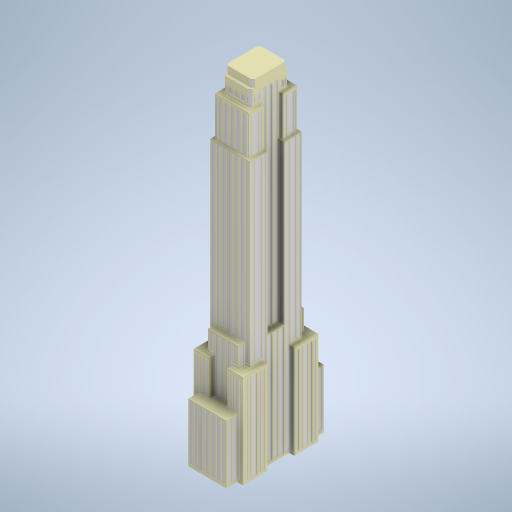
# Autodesk Inventor part: 樓底
Saved by Autodesk Inventor 2024.2 (Build 282272000, 272)
## iProperties
Created: 2024-05-30
Part Number: 樓底
Material: 一般
Document SubType Name: Modeling
Designer: User
Density: 1 g/cm^3
Appearance: 預設
Author: User
Autodesk Inventor part; units mm, degrees
(part 1 of 2)
sketch "草圖2" plane through (0, 0, 0) normal (0, 1, 0) x (-1, 0, 0)
  line L0 (36, 55) -> (36, -55)
  line L1 (36, -55) -> (-36, -55)
  line L2 (-36, -55) -> (-36, 55)
  line L3 (-36, 55) -> (36, 55)
  line L4 (36, 55) -> (-36, -55) construction
  line L5 (36, -55) -> (-36, 55) construction
  line L6 (36, 0) -> (36, -20)
  line L7 (36, 0) -> (36, 20)
  line L8 (36, 20) -> (36, -20)
  line L9 (36, -20) -> (29, -20)
  line L10 (29, -20) -> (29, 20)
  line L11 (29, 20) -> (36, 20)
  line L12 (0, 55) -> (0, -55)
  line L13 (-36, -20) -> (-29, -20)
  line L14 (-29, -20) -> (-29, 20)
  line L15 (-29, 20) -> (-36, 20)
  line L16 (0, 55) -> (13, 55)
  line L17 (0, 55) -> (-13, 55)
  line L18 (13, 55) -> (-13, 55)
  line L19 (-13, 55) -> (-13, 48)
  line L20 (-13, 48) -> (13, 48)
  line L21 (13, 48) -> (13, 55)
  line L22 (13, 0) -> (-13, 0)
  line L23 (-13, -55) -> (-13, -48)
  line L24 (-13, -48) -> (13, -48)
  line L25 (13, -48) -> (13, -55)
  point P0 (0, 0)
  dimension "d0" = 110
  dimension "d1" = 72
  dimension "d2" = 20
  dimension "d3" = 20
  dimension "d4" = 7
  dimension "d7" = 13
  dimension "d8" = 13
  dimension "d9" = 7
  constraints: 52 end point, 8 symmetric about line, 6 parallel, 5 midpoint, 4 point on line, 3 perpendicular, 2 collinear, 1 horizontal, 1 vertical
  measures "d0" distance of L0.start L0.end
  measures "d1" distance of L0.end L1.end
  measures "d2" distance of L6.start L6.end
  measures "d3" distance of L6.start L7.end
  measures "d4" distance of L6.end L9.end
  measures "d7" distance of L12.start L16.end
  measures "d8" distance of L12.start L17.end
  measures "d9" distance of L19.end L17.end
extrude "擠出2" add sketch "草圖2" along normal blind 137 contours L0 L11 L10 L9 L1 L25 L24 L12 L20 L21 L3 | L19 L20 L12 L24 L23 L1 L2 L13 L14 L15 L3
sketch "草圖3" plane through (0, 137, 0) normal (0, 1, 0) x (1, 0, 0)
  point P0 (0, 0)
sketch "草圖4" plane through (0, 137, 0) normal (0, 1, 0) x (1, 0, 0)
  line L0 (-29, -48) -> (29, -48)
  line L1 (29, -48) -> (29, 48)
  line L2 (29, 48) -> (-29, 48)
  line L3 (-29, 48) -> (-29, -48)
  line L4 (-29, -48) -> (29, 48) construction
  line L5 (29, -48) -> (-29, 48) construction
  line L6 (29, 48) -> (22, 48)
  line L7 (22, 48) -> (22, 38)
  line L8 (22, 38) -> (29, 38)
  line L9 (29, 38) -> (29, 48)
  line L10 (-29, 20) -> (-29, -20) projected
  line L11 (-29, 0) -> (29, 0)
  line L12 (0, 48) -> (0, -48)
  line L13 (-22, 48) -> (-22, 38)
  line L14 (-22, 38) -> (-29, 38)
  line L15 (29, 0) -> (-29, 0)
  line L16 (22, -48) -> (22, -38)
  line L17 (22, -38) -> (29, -38)
  line L18 (0, -48) -> (0, 48)
  line L19 (22, -48) -> (22, -38)
  line L20 (22, -38) -> (29, -38)
  line L21 (-22, -48) -> (-22, -38)
  line L22 (-22, -38) -> (-29, -38)
  point P0 (0, 0)
  dimension "d12" = 7
  dimension "d13" = 10
  constraints: 44 end point, 13 symmetric about line, 6 midpoint, 4 parallel, 2 perpendicular, 1 point on line
  measures "d12" distance of L1.end L6.end
  measures "d13" distance of L7.end L6.end
extrude "擠出3" add sketch "草圖4" along normal blind 29 contours L21 L22 L3 L11 L12 L0 | L12 L11 L1 L17 L16 L0 | L12 L2 L7 L8 L1 L11 | L11 L3 L14 L13 L2 L12
sketch "草圖5" plane through (0, 0, 0) normal (0, -1, 0) x (1, 0, 0)
  line L0 (0, -55) -> (28, -55)
  line L1 (36, -55) -> (13, -55) projected
  line L2 (0, -55) -> (-28, -55)
  line L3 (-13, -55) -> (-36, -55) projected
  line L4 (22, -48) -> (-22, -48) projected
  line L5 (13, -48) -> (-13, -48)
  line L6 (-13, -55) -> (-13, -48)
  line L7 (13, -48) -> (13, -55)
  line L8 (28, -55) -> (-28, -55)
  line L9 (-28, -55) -> (-28, -71)
  line L10 (-28, -71) -> (28, -71)
  line L11 (28, -71) -> (28, -55)
  line L12 (29, 38) -> (29, -38) projected
  line L13 (29, 0) -> (-29, 0)
  line L14 (-29, -38) -> (-29, 38) projected
  line L15 (0, 55) -> (-28, 55)
  line L16 (13, 48) -> (-13, 48)
  line L17 (-13, 55) -> (-13, 48)
  line L18 (13, 48) -> (13, 55)
  line L19 (-28, 55) -> (-28, 71)
  line L20 (-28, 71) -> (28, 71)
  line L21 (28, 71) -> (28, 55)
  line L22 (13, 55) -> (0, 55)
  line L23 (28, 55) -> (-28, 55)
  point P0 (0, 0)
  dimension "d16" = 28
  dimension "d17" = 28
  dimension "d18" = 16
  constraints: 38 end point, 9 symmetric about line, 4 point on line, 3 perpendicular, 2 collinear, 2 midpoint, 2 parallel, 1 horizontal
  measures "d16" distance of L0.start L0.end
  measures "d17" distance of L0.start L2.end
  measures "d18" distance of L9.end L2.end
extrude "擠出4" add sketch "草圖5" against normal blind 86
ref_plane "工作平面1" through (-22, 166, 0) normal (0, 0, 1) x (1, 0, 0)
ref_plane "工作平面3" through (0, 0, -55) normal (-1, 0, 0) x (0, 0, 1)
sketch "草圖12" plane through (0, 166, 0) normal (0, 1, 0) x (1, 0, 0)
  line L0 (29, -20) -> (29, 20) projected
  line L1 (29, 0) -> (29, 12)
  line L2 (29, 0) -> (29, -12)
  line L3 (29, -12) -> (29, 12)
  line L4 (29, 12) -> (20, 12)
  line L5 (20, 12) -> (20, -12)
  line L6 (20, -12) -> (29, -12)
  line L7 (0, -6) -> (0, 6)
  line L8 (-29, 0) -> (-29, 12)
  line L9 (-29, 0) -> (-29, -12)
  line L10 (-29, -12) -> (-29, 12)
  line L11 (-29, 12) -> (-20, 12)
  line L12 (-20, 12) -> (-20, -12)
  line L13 (-20, -12) -> (-29, -12)
  line L14 (-29, -38) -> (-29, -12)
  line L15 (-29, -12) -> (29, -12)
  line L16 (29, -12) -> (29, -38)
  line L17 (29, -38) -> (-29, -38)
  line L18 (-29, -20) -> (-36, -20) projected
  line L19 (-22, 38) -> (-29, 38) projected
  line L20 (-29, 12) -> (-29, 38)
  line L21 (-29, 38) -> (29, 38)
  line L22 (29, 38) -> (29, 12)
  line L23 (29, 12) -> (-29, 12)
  line L24 (-20, -12) -> (-20, 12)
  line L25 (-20, 12) -> (20, 12)
  line L26 (20, 12) -> (20, -12)
  line L27 (20, -12) -> (-20, -12)
  point P0 (0, 0)
  dimension "d89" = 12
  dimension "d90" = 12
  dimension "d91" = 9
  constraints: 50 end point, 8 parallel, 7 perpendicular, 6 symmetric about line, 2 point on line, 1 collinear, 1 midpoint, 1 vertical
  measures "d89" distance of L1.start L1.end
  measures "d90" distance of L1.start L2.end
  measures "d91" distance of L4.end L1.end
extrude "擠出9" add sketch "草圖12" along normal blind 232 contours L16 L17 L14 L13 L15 L6 L0 | L15 L12 L23 L5 | L4 L23 L11 L20 L19 L21 L22 L0
sketch "草圖13" plane through (0, 398, 0) normal (0, 1, 0) x (1, 0, 0)
  line L0 (-25, 35) -> (-25, -35)
  line L1 (-25, -35) -> (25, -35)
  line L2 (25, -35) -> (25, 35)
  line L3 (25, 35) -> (-25, 35)
  line L4 (-25, 35) -> (25, -35) construction
  line L5 (-25, -35) -> (25, 35) construction
  line L6 (-25, 0) -> (-20, 0)
  line L7 (-20, 0) -> (-20, -14)
  line L8 (-20, -14) -> (-25, -14)
  line L9 (-25, -14) -> (-25, 0)
  line L10 (-20, 0) -> (-25, 0)
  line L11 (-25, 0) -> (-25, 14)
  line L12 (-25, 14) -> (-20, 14)
  line L13 (-20, 14) -> (-20, 0)
  line L14 (-20, -12) -> (-20, 12) projected
  line L15 (0, 8.1433) -> (0, -10.4531)
  line L16 (-36, 55) -> (-36, 20) projected
  line L17 (25, 0) -> (20, 0)
  line L18 (20, 0) -> (20, -14)
  line L19 (20, -14) -> (25, -14)
  line L20 (25, -14) -> (25, 0)
  line L21 (20, 0) -> (25, 0)
  line L22 (25, 0) -> (25, 14)
  line L23 (25, 14) -> (20, 14)
  line L24 (20, 14) -> (20, 0)
  line L25 (20, -12) -> (20, 12)
  point P0 (0, 0)
  dimension "d94" = 70
  dimension "d95" = 50
  dimension "d96" = 5
  dimension "d97" = 14
  dimension "d98" = 14
  constraints: 48 end point, 8 symmetric about line, 7 parallel, 5 perpendicular, 3 midpoint, 1 vertical
  measures "d94" distance of L0.start L0.end
  measures "d95" distance of L1.end L0.end
  measures "d96" distance of L6.start L6.end
  measures "d97" distance of L6.end L7.end
  measures "d98" distance of L6.start L11.end
extrude "擠出10" add sketch "草圖13" along normal blind 58 contours L3 L2 L23 L24 L18 L19 L1 L0 L8 L7 L13 L12
sketch "草圖14" plane through (-20, 166, -12) normal (-1, 0, 0) x (0, 0, 1)
  line L0 (-23, 290) -> (-2, 290) projected
  line L1 (47, 232) -> (47, 290) projected
  line L2 (-23, 290) -> (47, 290)
  line L3 (26, 290) -> (-2, 290) projected
  line L4 (12, 290) -> (40.5, 290)
  line L5 (40.5, 290) -> (40.5, 324)
  line L6 (40.5, 324) -> (12, 324)
  line L7 (12, 324) -> (12, 290)
  line L8 (12, 324) -> (12, 290)
  line L9 (12, 290) -> (-16.5, 290)
  line L10 (-16.5, 290) -> (-16.5, 324)
  line L11 (-16.5, 324) -> (12, 324)
  line L12 (40.5, 324) -> (36.5, 324)
  line L13 (36.5, 324) -> (36.5, 313)
  line L14 (36.5, 313) -> (40.5, 313)
  line L15 (40.5, 313) -> (40.5, 324)
  line L16 (-16.5, 324) -> (-12.5, 324)
  line L17 (-12.5, 324) -> (-12.5, 313)
  line L18 (-12.5, 313) -> (-16.5, 313)
  line L19 (-16.5, 313) -> (-16.5, 324)
  point P0 (12, -166)
  dimension "d101" = 28.5
  dimension "d102" = 34
  dimension "d103" = 28.5
  dimension "d104" = 4
  dimension "d105" = 11
  dimension "d106" = 4
  constraints: 34 end point, 8 parallel, 5 perpendicular, 3 point on line, 1 horizontal, 1 midpoint
  measures "d101" distance of L4.start L4.end
  measures "d102" distance of L5.end L4.end
  measures "d103" distance of L4.start L9.end
  measures "d104" distance of L5.end L12.end
  measures "d105" distance of L13.end L12.end
  measures "d106" distance of L10.end L16.end
extrude "擠出11" add sketch "草圖14" against normal blind 40 contours L10 L18 L17 L11 L7 L2 L0 | L7 L6 L13 L14 L5 L2
sketch "草圖15" plane through (-36, 0, 20) normal (-1, 0, 0) x (0, 0, 1)
  line L0 (0, 137) -> (18, 137) projected
  line L1 (0, 137) -> (0, 132)
  line L2 (0, 0) -> (0, 137) projected
  line L3 (0, 132) -> (3.75, 132)
  line L4 (35, 86) -> (35, 137) projected
  line L5 (3.75, 132) -> (6.25, 132)
  line L6 (6.25, 132) -> (9.25, 132)
  line L7 (9.25, 132) -> (11.75, 132)
  line L8 (11.75, 132) -> (14.75, 132)
  line L9 (14.75, 132) -> (20.25, 132)
  line L10 (20.25, 132) -> (23.25, 132)
  line L11 (23.25, 132) -> (25.75, 132)
  line L12 (25.75, 132) -> (28.75, 132)
  line L13 (28.75, 132) -> (31.25, 132)
  line L14 (31.25, 132) -> (35, 132)
  line L15 (14.75, 132) -> (20.25, 132)
  line L16 (20.25, 132) -> (20.25, 132.25)
  line L17 (20, 132.25) -> (15, 132.25)
  line L18 (14.75, 132.25) -> (14.75, 132)
  arc A0 (18.25, 132) -> (16.75, 132) centre (17.5, 132) ccw
  line L19 (14.75, 132) -> (15, 132)
  arc A1 (15, 132.25) -> (14.75, 132) centre (15, 132) ccw
  line L20 (20.25, 132) -> (20, 132)
  arc A2 (20.25, 132) -> (20, 132.25) centre (20, 132) ccw
  line L21 (14.75, 132) -> (20.25, 132)
  line L22 (20.25, 132) -> (20.25, 4)
  line L23 (20.25, 4) -> (14.75, 4)
  line L24 (14.75, 4) -> (14.75, 132)
  line L25 (23.25, 132) -> (25.75, 132)
  line L26 (25.75, 132) -> (25.75, 4)
  line L27 (25.75, 4) -> (23.25, 4)
  line L28 (23.25, 4) -> (23.25, 132)
  line L29 (28.75, 132) -> (31.25, 132)
  line L30 (31.25, 132) -> (31.25, 4)
  line L31 (31.25, 4) -> (28.75, 4)
  line L32 (28.75, 4) -> (28.75, 132)
  line L33 (3.75, 132) -> (6.25, 132)
  line L34 (6.25, 132) -> (6.25, 4)
  line L35 (6.25, 4) -> (3.75, 4)
  line L36 (3.75, 4) -> (3.75, 132)
  line L37 (9.25, 132) -> (11.75, 132)
  line L38 (11.75, 132) -> (11.75, 4)
  line L39 (11.75, 4) -> (9.25, 4)
  line L40 (9.25, 4) -> (9.25, 132)
  line L41 (3.75, 132) -> (6.25, 132)
  line L42 (6.25, 132) -> (6.25, 132.25)
  line L43 (6.25, 132.25) -> (4, 132.25)
  line L44 (3.75, 132.25) -> (3.75, 132)
  line L45 (3.75, 132) -> (4, 132)
  line L46 (6.25, 132) -> (6, 132)
  arc A3 (4, 132.25) -> (4.25, 132) centre (4, 132) ccw
  arc A4 (5.75, 132) -> (6, 132.25) centre (6, 132) ccw
  line L47 (9.25, 132) -> (11.75, 132)
  line L48 (11.75, 132.25) -> (9.5, 132.25)
  arc A5 (9.5, 132.25) -> (9.75, 132) centre (9.5, 132) ccw
  arc A6 (11.25, 132) -> (11.5, 132.25) centre (11.5, 132) ccw
  line L49 (25.75, 132.25) -> (23.5, 132.25)
  arc A7 (23.5, 132.25) -> (23.75, 132) centre (23.5, 132) ccw
  arc A8 (25.25, 132) -> (25.5, 132.25) centre (25.5, 132) ccw
  line L50 (23.25, 132) -> (25.75, 132)
  line L51 (31.25, 132.25) -> (29, 132.25)
  arc A9 (29, 132.25) -> (29.25, 132) centre (29, 132) ccw
  arc A10 (30.75, 132) -> (31, 132.25) centre (31, 132) ccw
  line L52 (28.75, 132) -> (31.25, 132)
  point P0 (-20, 0)
  point P1 (18.2071, 132.25)
  point P2 (16.7929, 132.25)
  point P3 (14.75, 132)
  point P4 (34.25, 132)
  point P5 (11.75, 132)
  point P6 (9.25, 132)
  dimension "d109" = 5
  dimension "d110" = 3.75
  dimension "d111" = 2.5
  dimension "d112" = 3
  dimension "d113" = 2.5
  dimension "d114" = 3
  dimension "d115" = 5.5
  dimension "d116" = 3
  dimension "d117" = 2.5
  dimension "d118" = 3
  dimension "d119" = 2.5
  dimension "d120" = 0.25
  dimension "d121" = 1.5
  dimension "d122" = 0.25
  dimension "d123" = 0.25
  dimension "d124" = 128
  dimension "d125" = 128
  dimension "d126" = 128
  dimension "d127" = 128
  dimension "d128" = 128
  dimension "d131" = 0.25
  dimension "d132" = 0.25
  dimension "d133" = 0.25
  dimension "d136" = 5.5
  dimension "d143" = 14
  dimension "d150" = 5.5
  constraints: 100 end point, 26 point on line, 22 point on circle, 15 parallel, 11 centre point, 9 collinear, 9 perpendicular, 4 coincident, 3 horizontal, 3 tangent, 1 midpoint, 39 other
  measures "d109" distance of L0.start L1.end
  measures "d110" distance of L1.end L3.end
  measures "d111" distance of L3.end L5.end
  measures "d112" distance of L5.end L6.end
  measures "d113" distance of L6.end L7.end
  measures "d114" distance of L8.end L7.end
  measures "d115" distance of L8.end L9.end
  measures "d116" distance of L9.end L10.end
  measures "d117" distance of L10.end L11.end
  measures "d118" distance of L11.end L12.end
  measures "d119" distance of L12.end L13.end
  measures "d120" distance of L9.end L16.end
  measures "d121" diameter of A0
  measures "d122" distance of L8.end L19.end
  measures "d123" distance of L9.end L20.end
  measures "d124" distance of L9.end L22.end
  measures "d125" distance of L11.end L26.end
  measures "d126" distance of L13.end L30.end
  measures "d127" distance of L5.end L34.end
  measures "d128" distance of L7.end L38.end
  measures "d131" distance of L42.end L5.end
  measures "d132" distance of L3.end L45.end
  measures "d133" distance of L5.end L46.end
  measures "d136" distance of L3.end L47.start
  measures "d143" distance of L48.start L49.start
  measures "d150" distance of L49.start L51.start
extrude "擠出12" cut sketch "草圖15" against normal blind 0.6 contours A3 L43 A4 L5 | A3 L5 A4 L34 L35 L36 | A9 L51 A10 L13 | L13 A9 | A9 L13 A10 L30 L31 L32 | A7 L49 A8 L11 | L11 A7 | A7 L11 A8 L26 L27 L28 | A1 L17 A0 L9 | L9 L22 L23 L24 | A5 L48 A6 L7 | L7 A5 | A5 L7 A6 L38 L39 L40 | L5 A3 | L5 A4 | L7 A6 | A0 L17 L9 | A0 L17 | A0 L17 A2 L9 | L11 A8 | L13 A10
sketch "草圖16" plane through (-29, 0, -20) normal (-1, 0, 0) x (0, 0, 1)
  line L0 (0, 0) -> (0.25, 0)
  line L1 (0.25, 0) -> (5.75, 0)
  line L2 (5.75, 0) -> (8.75, 0)
  line L3 (8.75, 0) -> (14.25, 0)
  line L4 (14.25, 0) -> (17.25, 0)
  line L5 (17.25, 0) -> (22.75, 0)
  line L6 (22.75, 0) -> (25.75, 0)
  line L7 (25.75, 0) -> (31.25, 0)
  line L8 (31.25, 0) -> (34.25, 0)
  line L9 (34.25, 0) -> (39.75, 0)
  line L10 (40, 0) -> (75, 0) projected
  line L11 (39.75, 0) -> (40, 0)
  line L12 (17.25, 0) -> (22.75, 0)
  line L13 (22.75, 0) -> (22.75, 164)
  line L14 (22.75, 164) -> (17.25, 164)
  line L15 (17.25, 164) -> (17.25, 0)
  line L16 (0, 0) -> (40, 0) projected
  line L17 (25.75, 0) -> (31.25, 0)
  line L18 (31.25, 0) -> (31.25, 164)
  line L19 (31.25, 164) -> (25.75, 164)
  line L20 (25.75, 164) -> (25.75, 0)
  line L21 (8.75, 0) -> (14.25, 0)
  line L22 (14.25, 0) -> (14.25, 164)
  line L23 (14.25, 164) -> (8.75, 164)
  line L24 (8.75, 164) -> (8.75, 0)
  line L25 (34.25, 0) -> (39.75, 0)
  line L26 (39.75, 0) -> (39.75, 396)
  line L27 (39.75, 396) -> (34.25, 396)
  line L28 (34.25, 396) -> (34.25, 0)
  line L29 (5.75, 0) -> (0.25, 0)
  line L30 (0.25, 0) -> (0.25, 396)
  line L31 (0.25, 396) -> (5.75, 396)
  line L32 (5.75, 396) -> (5.75, 0)
  line L33 (0.25, 0) -> (0.25, 4)
  line L34 (0.25, 4) -> (39.75, 4)
  line L35 (8.75, 164) -> (14.25, 164)
  line L36 (14.25, 164) -> (14.25, 164.25)
  line L37 (14.25, 164.25) -> (8.75, 164.25)
  line L38 (8.75, 164.25) -> (8.75, 164)
  circle A0 centre (11.5, 164) radius 0.75
  line L39 (22.75, 164) -> (22.75, 164.25)
  line L40 (22.75, 164.25) -> (17.25, 164.25)
  line L41 (17.25, 164.25) -> (17.25, 164)
  line L42 (22.75, 164) -> (17.25, 164)
  line L43 (17.25, 164) -> (22.75, 164)
  circle A1 centre (20, 164) radius 0.75
  line L44 (31.25, 164) -> (31.25, 164.25)
  line L45 (31.25, 164.25) -> (25.75, 164.25)
  line L46 (25.75, 164.25) -> (25.75, 164)
  line L47 (31.25, 164) -> (25.75, 164)
  line L48 (25.75, 164) -> (31.25, 164)
  circle A2 centre (28.5, 164) radius 0.75
  line L49 (34.25, 396) -> (39.75, 396)
  line L50 (39.75, 396) -> (39.75, 396.25)
  line L51 (39.75, 396.25) -> (34.25, 396.25)
  line L52 (34.25, 396.25) -> (34.25, 396)
  circle A3 centre (37, 396) radius 0.75
  line L53 (34.25, 396) -> (34.5, 396)
  line L54 (39.75, 396) -> (39.5, 396)
  circle A4 centre (34.5, 396) radius 0.25
  circle A5 centre (39.5, 396) radius 0.25
  line L55 (5.75, 396) -> (0.25, 396)
  line L56 (0.25, 396) -> (0.5, 396)
  line L57 (0.25, 396.25) -> (0.25, 396)
  circle A6 centre (0.5, 396) radius 0.25
  line L58 (0.25, 396) -> (5.75, 396)
  line L59 (5.75, 396.25) -> (0.25, 396.25)
  line L60 (5.75, 396) -> (5.75, 396.25)
  circle A7 centre (5.5, 396) radius 0.25
  circle A8 centre (3, 396) radius 0.75
  line L61 (5.75, 396) -> (5.5, 396)
  line L62 (8.75, 164) -> (9, 164)
  line L63 (14.25, 164) -> (14, 164)
  circle A9 centre (9, 164) radius 0.25
  circle A10 centre (14, 164) radius 0.25
  circle A11 centre (17.5, 164) radius 0.25
  circle A12 centre (22.5, 164) radius 0.25
  circle A13 centre (26, 164) radius 0.25
  circle A14 centre (31, 164) radius 0.25
  point P0 (34.25, 4)
  point P1 (25.75, 4)
  point P2 (31.25, 4)
  point P3 (17.25, 4)
  point P4 (22.75, 4)
  point P5 (8.75, 4)
  point P6 (14.25, 4)
  point P7 (5.75, 4)
  point P8 (26, 164.25)
  point P9 (31, 164.25)
  point P10 (29.2071, 164.25)
  point P11 (27.7929, 164.25)
  point P12 (22.5, 164.25)
  point P13 (20.7071, 164.25)
  point P14 (19.2929, 164.25)
  point P15 (17.5, 164.25)
  point P16 (14, 164.25)
  point P17 (12.2071, 164.25)
  point P18 (10.7929, 164.25)
  point P19 (9, 164.25)
  point P20 (8.75, 164)
  point P21 (39.5, 396.25)
  point P22 (37.7071, 396.25)
  point P23 (36.2929, 396.25)
  point P24 (34.5, 396.25)
  point P25 (2.2929, 396.25)
  point P26 (0.5, 396.25)
  point P27 (0.25, 396)
  point P28 (5.75, 396)
  point P29 (5.5, 396.25)
  point P30 (3.7071, 396.25)
  dimension "d164" = 0.25
  dimension "d165" = 5.5
  dimension "d166" = 3
  dimension "d167" = 5.5
  dimension "d168" = 3
  dimension "d169" = 5.5
  dimension "d170" = 3
  dimension "d171" = 5.5
  dimension "d172" = 3
  dimension "d173" = 5.5
  dimension "d174" = 164
  dimension "d175" = 164
  dimension "d176" = 164
  dimension "d177" = 396
  dimension "d178" = 396
  dimension "d179" = 4
  dimension "d182" = 0.25
  dimension "d183" = 1.5
  dimension "d186" = 8.5
  dimension "d191" = 0.25
  dimension "d192" = 1.5
  dimension "d193" = 0.25
  dimension "d194" = 0.25
  dimension "d197" = 34
  dimension "d202" = 0.25
  dimension "d203" = 0.25
  dimension "d206" = 8.5
  constraints: 124 end point, 17 point on line, 14 parallel, 12 horizontal, 10 centre point, 8 perpendicular, 6 coincident, 5 collinear, 2 midpoint, 2 tangent, 62 other
  measures "d164" distance of L0.start L0.end
  measures "d165" distance of L0.end L1.end
  measures "d166" distance of L1.end L2.end
  measures "d167" distance of L2.end L3.end
  measures "d168" distance of L3.end L4.end
  measures "d169" distance of L4.end L5.end
  measures "d170" distance of L5.end L6.end
  measures "d171" distance of L6.end L7.end
  measures "d172" distance of L7.end L8.end
  measures "d173" distance of L8.end L9.end
  measures "d174" distance of L13.end L5.end
  measures "d175" distance of L18.end L7.end
  measures "d176" distance of L22.end L3.end
  measures "d177" distance of L26.end L9.end
  measures "d178" distance of L0.end L30.end
  measures "d179" distance of L0.end L33.end
  measures "d182" distance of L36.end L22.end
  measures "d183" diameter of A0
  measures "d186" distance of L36.end L39.end
  measures "d191" distance of L50.end L26.end
  measures "d192" diameter of A3
  measures "d193" distance of L27.end L53.end
  measures "d194" distance of L26.end L54.end
  measures "d197" distance of L26.end L55.start
  measures "d202" distance of L23.end L62.end
  measures "d203" distance of L22.end L63.end
  measures "d206" distance of A9.centre A11.centre
extrude "擠出13" cut sketch "草圖16" against normal blind 0.6 contours L30 A6 L31 A8 A7 L32 L34 | A6 L31 | L31 A6 | L24 A9 L23 A0 A10 L22 L34 | A7 L31 | L31 A7 | A6 L59 A8 L31 | A9 L23 | L23 A9 | A7 L31 A8 L59 | A8 L59 L31 | L31 A8 | A8 L59 | L15 A11 L14 A1 A12 L13 L34 | A10 L23 | L23 A10 | A9 L37 A0 L23 | A11 L14 | L14 A11 | A10 L23 A0 L37 | A0 L37 L23 | L23 A0 | A0 L37 | L20 A13 L19 A2 A14 L18 L34 | A12 L14 | L14 A12 | A11 L40 A1 L14 | A13 L19 | L19 A13 | L14 A1 L40 A12 | A1 L40 L14 | L14 A1 | A1 L40 | L28 A4 L27 A3 A5 L26 L34 | A14 L19 | L19 A14 | A13 L45 A2 L19 | A4 L27 | L27 A4 | L19 A2 L45 A14 | A2 L45 L19 | L19 A2 | A2 L45 | A5 L27 | L27 A5 | A4 L51 A3 L27 | A5 L27 A3 L51 | A3 L51 L27 | L27 A3 | A3 L51
sketch "草圖17" plane through (-29, 0, 20) normal (0, 0, -1) x (-1, 0, 0)
  line L0 (0, 0) -> (7, 0) projected
  line L1 (0, 0) -> (0.7, 0)
  line L2 (0.7, 0) -> (6.2, 0)
  line L3 (6.2, 0) -> (7, 0)
  line L4 (0.7, 0) -> (6.2, 0)
  line L5 (6.2, 0) -> (6.2, 132)
  line L6 (6.2, 132) -> (0.7, 132)
  line L7 (0.7, 132) -> (0.7, 0)
  line L8 (0.7, 132) -> (6.2, 132)
  line L9 (6.2, 132) -> (6.2, 132.25)
  line L10 (6.2, 132.25) -> (0.7, 132.25)
  line L11 (0.7, 132.25) -> (0.7, 132)
  line L12 (0.7, 132) -> (3.45, 132)
  circle A0 centre (3.45, 132) radius 0.75
  line L13 (0.7, 132) -> (0.95, 132)
  line L14 (6.2, 132) -> (5.95, 132)
  circle A1 centre (0.95, 132) radius 0.25
  circle A2 centre (5.95, 132) radius 0.25
  line L15 (0.7, 0) -> (6.2, 0)
  line L16 (6.2, 0) -> (6.2, 4)
  line L17 (6.2, 4) -> (0.7, 4)
  line L18 (0.7, 4) -> (0.7, 0)
  point P0 (-29, 0)
  point P1 (2.7429, 132.25)
  point P2 (0.95, 132.25)
  point P3 (6.2, 132)
  point P4 (5.95, 132.25)
  point P5 (4.1571, 132.25)
  point P6 (0.7, 4)
  point P7 (6.2, 4)
  dimension "d211" = 0.7
  dimension "d212" = 5.5
  dimension "d213" = 132
  dimension "d214" = 0.25
  dimension "d215" = 2.75
  dimension "d216" = 1.5
  dimension "d217" = 0.25
  dimension "d218" = 0.25
  dimension "d229" = 4
  constraints: 36 end point, 6 parallel, 4 perpendicular, 4 point on line, 3 coincident, 3 collinear, 2 centre point, 1 midpoint, 1 tangent, 3 other
  measures "d211" distance of L0.start L1.end
  measures "d212" distance of L1.end L2.end
  measures "d213" distance of L5.end L2.end
  measures "d214" distance of L9.end L5.end
  measures "d215" distance of L6.end L12.end
  measures "d216" diameter of A0
  measures "d217" distance of L6.end L13.end
  measures "d218" distance of L5.end L14.end
  measures "d229" distance of L16.end L2.end
extrude "擠出14" cut sketch "草圖17" against normal blind 0.6 contours L7 A1 L6 A0 A2 L5 L17 | A1 L6 | L6 A1 | A2 L6 | L6 A2 | A1 L10 A0 L6 | A2 L6 A0 L10 | A0 L10 L6 | L6 A0 | A0 L10
sketch "草圖18" plane through (-36, 137, 55) normal (0, 0, 1) x (1, 0, 0)
  line L0 (8, -137) -> (8, -51) projected
  line L1 (8, -51) -> (23, -51) projected
  line L2 (23, -51) -> (23, 0) projected
  line L3 (0, 0) -> (23, 0) projected
  line L4 (0, -137) -> (0, 0) projected
  line L5 (0, -137) -> (8, -137) projected
  line L6 (0, -137) -> (3.2, -137)
  line L7 (3.2, -137) -> (5.7, -137)
  line L8 (5.7, -137) -> (8, -137)
  line L9 (8, -51) -> (8.2, -51)
  line L10 (8.2, -51) -> (10.7, -51)
  line L11 (10.7, -51) -> (13.2, -51)
  line L12 (13.2, -51) -> (15.7, -51)
  line L13 (15.7, -51) -> (18.2, -51)
  line L14 (18.2, -51) -> (20.7, -51)
  line L15 (20.7, -51) -> (23, -51)
  line L16 (3.2, -137) -> (5.7, -137)
  line L17 (5.7, -137) -> (5.7, -5)
  line L18 (5.7, -5) -> (3.2, -5)
  line L19 (3.2, -5) -> (3.2, -137)
  line L20 (10.7, -51) -> (8.2, -51)
  line L21 (8.2, -51) -> (8.2, -5)
  line L22 (8.2, -5) -> (10.7, -5)
  line L23 (10.7, -5) -> (10.7, -51)
  line L24 (13.2, -51) -> (15.7, -51)
  line L25 (15.7, -51) -> (15.7, -5)
  line L26 (15.7, -5) -> (13.2, -5)
  line L27 (13.2, -5) -> (13.2, -51)
  line L28 (18.2, -51) -> (20.7, -51)
  line L29 (20.7, -51) -> (20.7, -5)
  line L30 (20.7, -5) -> (18.2, -5)
  line L31 (18.2, -5) -> (18.2, -51)
  line L32 (8.2, -51) -> (20.7, -51)
  line L33 (20.7, -51) -> (20.7, -50)
  line L34 (20.7, -50) -> (8.2, -50)
  line L35 (8.2, -50) -> (8.2, -51)
  line L36 (3.2, -137) -> (5.7, -137)
  line L37 (5.7, -137) -> (5.7, -133)
  line L38 (5.7, -133) -> (3.2, -133)
  line L39 (3.2, -133) -> (3.2, -137)
  line L40 (3.2, -5) -> (5.7, -5)
  line L41 (5.7, -5) -> (5.7, -4.75)
  line L42 (5.7, -4.75) -> (3.2, -4.75)
  line L43 (3.2, -4.75) -> (3.2, -5)
  line L44 (3.2, -5) -> (3.45, -5)
  line L45 (5.7, -5) -> (5.45, -5)
  circle A0 centre (3.45, -5) radius 0.25
  circle A1 centre (5.45, -5) radius 0.25
  circle A2 centre (8.45, -5) radius 0.25
  line L46 (10.7, -4.75) -> (8.2, -4.75)
  circle A3 centre (10.45, -5) radius 0.25
  circle A4 centre (13.45, -5) radius 0.25
  line L47 (15.7, -4.75) -> (13.2, -4.75)
  circle A5 centre (15.45, -5) radius 0.25
  circle A6 centre (18.45, -5) radius 0.25
  line L48 (20.7, -4.75) -> (18.2, -4.75)
  circle A7 centre (20.45, -5) radius 0.25
  point P0 (36, -137)
  point P1 (8.2, -5)
  point P2 (10.7, -5)
  point P3 (13.2, -5)
  point P4 (15.7, -5)
  point P5 (18.2, -5)
  point P6 (20.7, -5)
  point P7 (18.2, -50)
  point P8 (20.7, -50)
  point P9 (20.45, -4.75)
  point P10 (18.45, -4.75)
  point P11 (13.2, -50)
  point P12 (15.7, -50)
  point P13 (15.45, -4.75)
  point P14 (13.45, -4.75)
  point P15 (10.7, -50)
  point P16 (10.45, -4.75)
  point P17 (8.45, -4.75)
  point P18 (5.45, -4.75)
  point P19 (3.45, -4.75)
  point P20 (3.2, -133)
  point P21 (5.7, -133)
  dimension "d221" = 3.2
  dimension "d222" = 2.5
  dimension "d223" = 0.2
  dimension "d224" = 2.5
  dimension "d225" = 2.5
  dimension "d226" = 2.5
  dimension "d227" = 2.5
  dimension "d228" = 2.5
  dimension "d230" = 132
  dimension "d231" = 1
  dimension "d232" = 4
  dimension "d233" = 0.25
  dimension "d234" = 0.25
  dimension "d235" = 0.25
  dimension "d238" = 5
  constraints: 86 end point, 14 parallel, 10 perpendicular, 10 point on line, 8 horizontal, 6 collinear, 2 coincident, 44 other
  measures "d221" distance of L4.start L6.end
  measures "d222" distance of L6.end L7.end
  measures "d223" distance of L0.end L9.end
  measures "d224" distance of L9.end L10.end
  measures "d225" distance of L10.end L11.end
  measures "d226" distance of L11.end L12.end
  measures "d227" distance of L12.end L13.end
  measures "d228" distance of L13.end L14.end
  measures "d230" distance of L17.end L7.end
  measures "d231" distance of L33.end L14.end
  measures "d232" distance of L37.end L7.end
  measures "d233" distance of L41.end L17.end
  measures "d234" distance of L18.end L44.end
  measures "d235" distance of L17.end L45.end
  measures "d238" distance of point (3.45, -5) point (8.45, -5)
extrude "擠出15" cut sketch "草圖18" against normal blind 0.6 contours L38 L19 A0 L18 A1 L17 | L21 A2 L22 A3 L23 L34 | A1 L18 | L18 A1 | A2 L22 | L22 A2 | A0 L18 | L18 A0 | A1 L18 A0 L42 | L27 A4 L26 A5 L25 L34 | A3 L22 | L22 A3 | A2 L46 A3 L22 | A4 L26 | L26 A4 | L31 A6 L30 A7 L29 L34 | A5 L26 | L26 A5 | A4 L47 A5 L26 | A6 L30 | L30 A6 | A7 L30 | L30 A7 | A6 L48 A7 L30
sketch "草圖19" plane through (-22, 166, 48) normal (0, 0, 1) x (1, 0, 0)
  line L0 (9, -80) -> (35, -80) projected
  line L1 (35, -80) -> (35, -29) projected
  line L2 (44, -29) -> (35, -29) projected
  line L3 (44, -29) -> (44, 0) projected
  line L4 (0, 0) -> (44, 0) projected
  line L5 (0, -29) -> (0, 0) projected
  line L6 (9, -29) -> (0, -29) projected
  line L7 (9, -80) -> (9, -29) projected
  line L8 (0, -29) -> (2.25, -29)
  line L9 (2.25, -29) -> (7.75, -29)
  line L10 (7.75, -29) -> (9, -29)
  line L11 (9, -80) -> (10.75, -80)
  line L12 (10.75, -80) -> (16.25, -80)
  line L13 (16.25, -80) -> (19.25, -80)
  line L14 (19.25, -80) -> (24.75, -80)
  line L15 (24.75, -80) -> (27.75, -80)
  line L16 (27.75, -80) -> (33.25, -80)
  line L17 (33.25, -80) -> (35, -80)
  line L18 (35, -29) -> (36.25, -29)
  line L19 (36.25, -29) -> (41.75, -29)
  line L20 (44, -29) -> (44, 0) projected
  line L21 (41.75, -29) -> (44, -29)
  line L22 (41.75, -29) -> (44, -29)
  line L23 (2.25, -29) -> (7.75, -29)
  line L24 (7.75, -29) -> (7.75, -2)
  line L25 (2.25, -2) -> (2.25, -29)
  line L26 (0, -29) -> (9, -29) projected
  line L27 (2.25, -29) -> (7.75, -29)
  line L28 (7.75, -29) -> (7.75, -26)
  line L29 (7.75, -26) -> (2.25, -26)
  line L30 (2.25, -26) -> (2.25, -29)
  line L31 (10.75, -80) -> (16.25, -80)
  line L32 (16.25, -80) -> (16.25, -2)
  line L33 (16.25, -2) -> (10.75, -2)
  line L34 (10.75, -2) -> (10.75, -80)
  line L35 (10.75, -80) -> (16.25, -80)
  line L36 (16.25, -80) -> (16.25, -79)
  line L37 (16.25, -79) -> (10.75, -79)
  line L38 (10.75, -79) -> (10.75, -80)
  line L39 (19.25, -80) -> (24.75, -80)
  line L40 (24.75, -80) -> (24.75, -2)
  line L41 (24.75, -2) -> (19.25, -2)
  line L42 (19.25, -2) -> (19.25, -80)
  line L43 (27.75, -80) -> (33.25, -80)
  line L44 (33.25, -80) -> (33.25, -2)
  line L45 (33.25, -2) -> (27.75, -2)
  line L46 (27.75, -2) -> (27.75, -80)
  line L47 (19.25, -80) -> (24.75, -80)
  line L48 (24.75, -80) -> (24.75, -79)
  line L49 (24.75, -79) -> (19.25, -79)
  line L50 (19.25, -79) -> (19.25, -80)
  line L51 (27.75, -80) -> (33.25, -80)
  line L52 (33.25, -80) -> (33.25, -79)
  line L53 (33.25, -79) -> (27.75, -79)
  line L54 (27.75, -79) -> (27.75, -80)
  line L55 (36.25, -29) -> (41.75, -29)
  line L56 (41.75, -29) -> (41.75, -2)
  line L57 (41.75, -2) -> (36.25, -2)
  line L58 (36.25, -2) -> (36.25, -29)
  line L59 (36.25, -29) -> (41.75, -29)
  line L60 (41.75, -29) -> (41.75, -26)
  line L61 (41.75, -26) -> (36.25, -26)
  line L62 (36.25, -26) -> (36.25, -29)
  line L63 (7.75, -2) -> (7.75, -1.75)
  line L64 (2.25, -1.75) -> (2.25, -2)
  arc A0 (5.7071, -1.75) -> (4.2929, -1.75) centre (5, -2) ccw
  line L65 (2.25, -2) -> (2.5, -2)
  arc A1 (2.5, -1.75) -> (2.25, -2) centre (2.5, -2) ccw
  line L66 (7.75, -2) -> (7.5, -2)
  arc A2 (7.75, -2) -> (7.5, -1.75) centre (7.5, -2) ccw
  line L67 (2.75, -2) -> (2.25, -2)
  line L68 (7.75, -2) -> (7.25, -2)
  line L69 (7.75, -1.75) -> (5.7071, -1.75)
  line L70 (4.2929, -1.75) -> (2.25, -1.75)
  line L71 (4.25, -2) -> (5.75, -2)
  line L72 (7.25, -2) -> (7.75, -2)
  arc A3 (11, -1.75) -> (10.75, -2) centre (11, -2) ccw
  line L73 (12.7929, -1.75) -> (10.75, -1.75)
  arc A4 (14.2071, -1.75) -> (12.7929, -1.75) centre (13.5, -2) ccw
  line L74 (16.25, -1.75) -> (14.2071, -1.75)
  arc A5 (16.25, -2) -> (16, -1.75) centre (16, -2) ccw
  arc A6 (19.5, -1.75) -> (19.25, -2) centre (19.5, -2) ccw
  line L75 (21.2929, -1.75) -> (19.25, -1.75)
  arc A7 (22.7071, -1.75) -> (21.2929, -1.75) centre (22, -2) ccw
  line L76 (24.75, -1.75) -> (22.7071, -1.75)
  arc A8 (24.75, -2) -> (24.5, -1.75) centre (24.5, -2) ccw
  arc A9 (28, -1.75) -> (27.75, -2) centre (28, -2) ccw
  line L77 (29.7929, -1.75) -> (27.75, -1.75)
  arc A10 (31.2071, -1.75) -> (29.7929, -1.75) centre (30.5, -2) ccw
  line L78 (33.25, -1.75) -> (31.2071, -1.75)
  arc A11 (33.25, -2) -> (33, -1.75) centre (33, -2) ccw
  arc A12 (36.5, -1.75) -> (36.25, -2) centre (36.5, -2) ccw
  line L79 (38.2929, -1.75) -> (36.25, -1.75)
  arc A13 (39.7071, -1.75) -> (38.2929, -1.75) centre (39, -2) ccw
  line L80 (41.75, -1.75) -> (39.7071, -1.75)
  arc A14 (41.75, -2) -> (41.5, -1.75) centre (41.5, -2) ccw
  point P0 (22, -166)
  point P1 (11.25, -2)
  point P2 (12.75, -2)
  point P3 (14.25, -2)
  point P4 (15.75, -2)
  point P5 (19.75, -2)
  point P6 (21.25, -2)
  point P7 (22.75, -2)
  point P8 (24.25, -2)
  point P9 (28.25, -2)
  point P10 (29.75, -2)
  point P11 (31.25, -2)
  point P12 (32.75, -2)
  point P13 (36.75, -2)
  point P14 (38.25, -2)
  point P15 (39.75, -2)
  point P16 (41.25, -2)
  point P17 (41.75, -2)
  point P18 (36.25, -2)
  point P19 (36.25, -26)
  point P20 (41.75, -26)
  point P21 (27.75, -2)
  point P22 (33.25, -2)
  point P23 (24.75, -2)
  point P24 (19.25, -2)
  point P25 (16.25, -2)
  point P26 (10.75, -2)
  point P27 (2.25, -26)
  point P28 (7.75, -26)
  dimension "d245" = 2.25
  dimension "d246" = 5.5
  dimension "d247" = 1.75
  dimension "d248" = 5.5
  dimension "d249" = 3
  dimension "d250" = 5.5
  dimension "d251" = 3
  dimension "d252" = 5.5
  dimension "d253" = 1.25
  dimension "d254" = 5.5
  dimension "d255" = 27
  dimension "d256" = 3
  dimension "d257" = 1
  dimension "d258" = 1
  dimension "d259" = 1
  dimension "d260" = 3
  dimension "d261" = 0.25
  dimension "d262" = 1.5
  dimension "d263" = 0.25
  dimension "d264" = 0.25
  dimension "d267" = 8.5
  constraints: 142 end point, 50 point on circle, 26 parallel, 20 point on line, 16 collinear, 15 centre point, 15 perpendicular, 6 coincident, 2 midpoint, 1 horizontal, 83 other
  measures "d245" distance of L5.start L8.end
  measures "d246" distance of L8.end L9.end
  measures "d247" distance of L0.start L11.end
  measures "d248" distance of L11.end L12.end
  measures "d249" distance of L12.end L13.end
  measures "d250" distance of L13.end L14.end
  measures "d251" distance of L14.end L15.end
  measures "d252" distance of L15.end L16.end
  measures "d253" distance of L1.end L18.end
  measures "d254" distance of L18.end L19.end
  measures "d255" distance of L24.end L9.end
  measures "d256" distance of L28.end L9.end
  measures "d257" distance of L36.end L12.end
  measures "d258" distance of L48.end L14.end
  measures "d259" distance of L52.end L16.end
  measures "d260" distance of L60.end L19.end
  measures "d261" distance of L63.end L24.end
  measures "d262" diameter of A0
  measures "d263" distance of L25.start L65.end
  measures "d264" distance of L24.end L66.end
  measures "d267" distance of A1.centre A3.centre
extrude "擠出16" cut sketch "草圖19" against normal blind 0.6 contours L34 L33 L32 L37 | A3 L73 A4 L74 A5 L33 | L29 L25 A1 L70 A0 L69 A2 L24 | L42 L41 L40 L49 | A6 L75 A7 L76 A8 L41 | L46 L45 L44 L53 | A9 L77 A10 L78 A11 L45 | L61 L58 L57 L56 | L57 A12 L79 A13 L80 A14
sketch "草圖20" plane through (-22, 137, 38) normal (-1, 0, 0) x (0, 0, 1)
  line L0 (10, 0) -> (0, 0) projected
  line L1 (0, 0) -> (2.25, 0)
  line L2 (2.25, 0) -> (7.75, 0)
  line L3 (7.75, 0) -> (10, 0)
  line L4 (2.25, 0) -> (7.75, 0)
  line L5 (7.75, 0) -> (7.75, 27)
  line L6 (2.25, 27) -> (2.25, 0)
  line L7 (7.75, 27) -> (7.75, 27.25)
  line L8 (7.75, 27.25) -> (2.25, 27.25)
  line L9 (2.25, 27.25) -> (2.25, 27)
  line L10 (2.25, 27) -> (2.5, 27)
  line L11 (7.75, 27) -> (7.5, 27)
  circle A0 centre (2.5, 27) radius 0.25
  circle A1 centre (7.5, 27) radius 0.25
  arc A2 (5.75, 27) -> (4.25, 27) centre (5, 27) ccw
  line L12 (2.75, 27) -> (2.25, 27)
  line L13 (2.25, 27) -> (2.75, 27)
  line L14 (7.25, 27) -> (7.75, 27)
  line L15 (7.75, 27) -> (7.25, 27)
  line L16 (5.75, 27) -> (4.25, 27)
  line L17 (2.25, 0) -> (7.75, 0)
  line L18 (7.75, 0) -> (7.75, 3)
  line L19 (7.75, 3) -> (2.25, 3)
  line L20 (2.25, 3) -> (2.25, 0)
  point P0 (-38, -137)
  point P1 (2.5, 27.25)
  point P2 (7.5, 27.25)
  point P3 (4.2929, 27.25)
  point P4 (5.7071, 27.25)
  point P5 (2.25, 3)
  point P6 (7.75, 3)
  dimension "d274" = 2.25
  dimension "d275" = 5.5
  dimension "d276" = 2.25
  dimension "d277" = 27
  dimension "d278" = 0.25
  dimension "d279" = 0.25
  dimension "d280" = 0.25
  dimension "d281" = 1.5
  dimension "d403" = 3
  constraints: 40 end point, 9 parallel, 6 perpendicular, 6 point on circle, 3 centre point, 3 collinear, 2 coincident, 2 midpoint, 2 point on line
  measures "d274" distance of L0.end L1.end
  measures "d275" distance of L1.end L2.end
  measures "d276" distance of L2.end L0.start
  measures "d277" distance of L5.end L2.end
  measures "d278" distance of L7.end L5.end
  measures "d279" distance of L6.start L10.end
  measures "d280" distance of L5.end L11.end
  measures "d281" diameter of A2
  measures "d403" distance of L18.end L2.end
extrude "擠出17" cut sketch "草圖20" against normal blind 0.6 contours L19 L6 A0 L8 A2 L16 A1 L5 | A1 L14 L11 | L11 L14 A1 | A0 L12 L10 | L10 L12 A0 | A2 L16 L8 | L8 A2
sketch "草圖21" plane through (22, 137, 38) normal (0, 0, 1) x (1, 0, 0)
  line L0 (7, 0) -> (0, 0) projected
  line L1 (7, 0) -> (7, 261) projected
  line L2 (-51, 261) -> (7, 261) projected
  line L3 (-51, 0) -> (-51, 261) projected
  line L4 (-44, 0) -> (-51, 0) projected
  line L5 (-44, 0) -> (-44, 29) projected
  line L6 (0, 29) -> (-44, 29) projected
  line L7 (0, 0) -> (0, 29) projected
  line L8 (-51, 29) -> (-51, 261) projected
  line L9 (-2, 29) -> (7, 29) projected
  line L10 (-44, 29) -> (-41.75, 29)
  line L11 (-41.75, 29) -> (-36.25, 29)
  line L12 (-36.25, 29) -> (-33.25, 29)
  line L13 (-33.25, 29) -> (-27.75, 29)
  line L14 (-27.75, 29) -> (-24.75, 29)
  line L15 (-24.75, 29) -> (-19.25, 29)
  line L16 (-19.25, 29) -> (-16.25, 29)
  line L17 (-16.25, 29) -> (-10.75, 29)
  line L18 (-10.75, 29) -> (-7.75, 29)
  line L19 (-7.75, 29) -> (-2.25, 29)
  line L20 (-2.25, 29) -> (0, 29)
  line L21 (6.25, 29) -> (7, 29)
  line L22 (0, 29) -> (5.5, 29)
  line L23 (5.5, 29) -> (7, 29)
  line L24 (5.5, 29) -> (7, 29)
  line L25 (-44, 29) -> (-49.5, 29)
  line L26 (-49.5, 29) -> (-51, 29)
  line L27 (0, 29) -> (5.5, 29)
  line L28 (5.5, 29) -> (5.5, 3)
  line L29 (5.5, 3) -> (0, 3)
  line L30 (0, 3) -> (0, 29)
  line L31 (-49.5, 29) -> (-44, 29)
  line L32 (-44, 29) -> (-44, 3)
  line L33 (-44, 3) -> (-49.5, 3)
  line L34 (-49.5, 3) -> (-49.5, 29)
  line L35 (-42, 29) -> (-51, 29) projected
  line L36 (5.5, 3) -> (0, 3)
  line L37 (0, 3) -> (0, 259)
  line L38 (0, 259) -> (5.5, 259)
  line L39 (5.5, 259) -> (5.5, 3)
  line L40 (-49.5, 29) -> (-44, 29)
  line L41 (-44, 29) -> (-44, 259)
  line L42 (-44, 259) -> (-49.5, 259)
  line L43 (-49.5, 259) -> (-49.5, 29)
  line L44 (-41.75, 29) -> (-36.25, 29)
  line L45 (-36.25, 29) -> (-36.25, 259)
  line L46 (-36.25, 259) -> (-41.75, 259)
  line L47 (-41.75, 259) -> (-41.75, 29)
  line L48 (-44, 29) -> (0, 29) projected
  line L49 (-33.25, 259) -> (-33.25, 29)
  line L50 (-27.75, 259) -> (-33.25, 259)
  line L51 (-27.75, 29) -> (-27.75, 259)
  line L52 (-24.75, 259) -> (-24.75, 29)
  line L53 (-19.25, 259) -> (-24.75, 259)
  line L54 (-19.25, 29) -> (-19.25, 259)
  line L55 (-16.25, 259) -> (-16.25, 29)
  line L56 (-10.75, 259) -> (-16.25, 259)
  line L57 (-10.75, 29) -> (-10.75, 259)
  line L58 (-7.75, 259) -> (-7.75, 29)
  line L59 (-2.25, 259) -> (-7.75, 259)
  line L60 (-2.25, 29) -> (-2.25, 259)
  line L61 (-36.25, 259) -> (-36.25, 259.25)
  line L62 (-36.25, 259.25) -> (-41.75, 259.25)
  line L63 (-41.75, 259.25) -> (-41.75, 259)
  line L64 (-41.75, 259) -> (-41.5, 259)
  line L65 (-36.25, 259) -> (-36.5, 259)
  arc A0 (-41.5, 259.25) -> (-41.75, 259) centre (-41.5, 259) ccw
  arc A1 (-36.25, 259) -> (-36.5, 259.25) centre (-36.5, 259) ccw
  arc A2 (-38.2929, 259.25) -> (-39.7071, 259.25) centre (-39, 259) ccw
  line L66 (-41.75, 259) -> (-41.25, 259)
  line L67 (-36.75, 259) -> (-36.25, 259)
  arc A3 (-33, 259.25) -> (-33.25, 259) centre (-33, 259) ccw
  line L68 (-27.75, 259.25) -> (-33.25, 259.25)
  arc A4 (-29.7929, 259.25) -> (-31.2071, 259.25) centre (-30.5, 259) ccw
  arc A5 (-27.75, 259) -> (-28, 259.25) centre (-28, 259) ccw
  arc A6 (-24.5, 259.25) -> (-24.75, 259) centre (-24.5, 259) ccw
  line L69 (-19.25, 259.25) -> (-24.75, 259.25)
  arc A7 (-21.2929, 259.25) -> (-22.7071, 259.25) centre (-22, 259) ccw
  arc A8 (-19.25, 259) -> (-19.5, 259.25) centre (-19.5, 259) ccw
  arc A9 (-16, 259.25) -> (-16.25, 259) centre (-16, 259) ccw
  line L70 (-10.75, 259.25) -> (-16.25, 259.25)
  arc A10 (-12.7929, 259.25) -> (-14.2071, 259.25) centre (-13.5, 259) ccw
  arc A11 (-10.75, 259) -> (-11, 259.25) centre (-11, 259) ccw
  arc A12 (-7.5, 259.25) -> (-7.75, 259) centre (-7.5, 259) ccw
  line L71 (-2.25, 259.25) -> (-7.75, 259.25)
  arc A13 (-4.2929, 259.25) -> (-5.7071, 259.25) centre (-5, 259) ccw
  arc A14 (-2.25, 259) -> (-2.5, 259.25) centre (-2.5, 259) ccw
  line L72 (5.5, 259.25) -> (0, 259.25)
  arc A15 (3.4571, 259.25) -> (2.0429, 259.25) centre (2.75, 259) ccw
  arc A16 (0.25, 259.25) -> (0, 259) centre (0.25, 259) ccw
  arc A17 (5.5, 259) -> (5.25, 259.25) centre (5.25, 259) ccw
  line L73 (-44, 259) -> (-49.5, 259)
  line L74 (-44, 259) -> (-44, 259.25)
  line L75 (-44, 259.25) -> (-49.5, 259.25)
  line L76 (-49.5, 259.25) -> (-49.5, 259)
  line L77 (-44, 259) -> (-44.25, 259)
  arc A18 (-44, 259) -> (-44.25, 259.25) centre (-44.25, 259) ccw
  line L78 (-44.5, 259) -> (-44, 259)
  arc A19 (-46.0429, 259.25) -> (-47.4571, 259.25) centre (-46.75, 259) ccw
  line L79 (-49.5, 259) -> (-49, 259)
  arc A20 (-49.25, 259.25) -> (-49.5, 259) centre (-49.25, 259) ccw
  line L80 (-49.5, 259) -> (-49.25, 259)
  line L81 (-41.75, 29) -> (-36.25, 29)
  line L82 (-36.25, 29) -> (-36.25, 30)
  line L83 (-36.25, 30) -> (-41.75, 30)
  line L84 (-41.75, 30) -> (-41.75, 29)
  line L85 (-33.25, 29) -> (-27.75, 29)
  line L86 (-27.75, 29) -> (-27.75, 30)
  line L87 (-33.25, 29) -> (-27.75, 29)
  line L88 (-33.25, 29) -> (-27.75, 29)
  line L89 (-33.25, 30) -> (-33.25, 29)
  line L90 (-27.75, 30) -> (-33.25, 30)
  line L91 (-24.75, 29) -> (-19.25, 29)
  line L92 (-19.25, 29) -> (-19.25, 30)
  line L93 (-24.75, 29) -> (-19.25, 29)
  line L94 (-24.75, 29) -> (-19.25, 29)
  line L95 (-24.75, 30) -> (-24.75, 29)
  line L96 (-19.25, 30) -> (-24.75, 30)
  line L97 (-16.25, 29) -> (-10.75, 29)
  line L98 (-10.75, 29) -> (-10.75, 30)
  line L99 (-16.25, 29) -> (-10.75, 29)
  line L100 (-16.25, 29) -> (-10.75, 29)
  line L101 (-16.25, 30) -> (-16.25, 29)
  line L102 (-10.75, 30) -> (-16.25, 30)
  line L103 (-7.75, 29) -> (-2.25, 29)
  line L104 (-2.25, 29) -> (-2.25, 30)
  line L105 (-7.75, 29) -> (-2.25, 29)
  line L106 (-7.75, 29) -> (-2.25, 29)
  line L107 (-7.75, 30) -> (-7.75, 29)
  line L108 (-2.25, 30) -> (-7.75, 30)
  line L109 (-41.75, 29) -> (-36.25, 29)
  point P0 (-22, -137)
  point P1 (0, 259)
  point P2 (0, 3)
  point P3 (5.5, 29)
  point P4 (5.5, 259)
  point P5 (-7.75, 30)
  point P6 (-16.25, 30)
  point P7 (-24.75, 30)
  point P8 (-33.25, 30)
  point P9 (-41.75, 30)
  dimension "d286" = 2.25
  dimension "d287" = 5.5
  dimension "d288" = 3
  dimension "d289" = 5.5
  dimension "d290" = 3
  dimension "d291" = 5.5
  dimension "d292" = 3
  dimension "d293" = 5.5
  dimension "d294" = 3
  dimension "d295" = 5.5
  dimension "d296" = 2.25
  dimension "d298" = 5.5
  dimension "d299" = 5.5
  dimension "d300" = 26
  dimension "d301" = 26
  dimension "d302" = 256
  dimension "d305" = 8.5
  dimension "d310" = 0.25
  dimension "d311" = 0.25
  dimension "d312" = 0.25
  dimension "d313" = 1.5
  dimension "d316" = 8.5
  dimension "d323" = 7.75
  dimension "d330" = 7.75
  dimension "d335" = 1
  dimension "d338" = 8.5
  constraints: 196 end point, 42 point on circle, 35 point on line, 21 centre point, 15 parallel, 14 collinear, 10 perpendicular, 7 horizontal, 4 coincident, 4 midpoint, 184 other
  measures "d286" distance of L10.start L10.end
  measures "d287" distance of L10.end L11.end
  measures "d288" distance of L11.end L12.end
  measures "d289" distance of L12.end L13.end
  measures "d290" distance of L13.end L14.end
  measures "d291" distance of L14.end L15.end
  measures "d292" distance of L15.end L16.end
  measures "d293" distance of L16.end L17.end
  measures "d294" distance of L17.end L18.end
  measures "d295" distance of L18.end L19.end
  measures "d296" distance of L19.end L20.end
  measures "d298" distance of L20.end L22.end
  measures "d299" distance of L10.start L25.end
  measures "d300" distance of L22.end L28.end
  measures "d301" distance of L10.start L32.end
  measures "d302" distance of L29.end L37.end
  measures "d305" distance of L46.end L49.start
  measures "d310" distance of L61.end L45.end
  measures "d311" distance of L46.end L64.end
  measures "d312" distance of L45.end L65.end
  measures "d313" diameter of A2
  measures "d316" distance of A0.centre A3.centre
  measures "d323" distance of L71.start L72.start
  measures "d330" distance of L45.end L73.start
  measures "d335" distance of L82.end L81.end
  measures "d338" distance of L11.end L85.end
extrude "擠出18" cut sketch "草圖21" against normal blind 0.6 contours L7 L9 L28 L29 | L37 L38 L39 L9 | A16 L72 A17 L38 | L43 L42 L41 L25 | L25 L5 L33 L34 | L108 L58 L59 L60 | A15 L72 | A20 L75 A18 L42 | L59 A12 L71 A14 | L102 L55 L56 L57 | A19 L75 | L56 A9 L70 A11 | L71 A13 | L47 L46 L45 L83 | L96 L52 L53 L54 | A0 L62 A1 L46 | L53 A6 L69 A8 | L70 A10 | L49 L50 L51 L90 | A3 L68 A5 L50 | A2 L62 | L69 A7 | A4 L68
sketch "草圖22" plane through (-29, 0, -20) normal (-1, 0, 0) x (0, 0, 1)
  line L0 (8, 166) -> (32, 166) projected
  line L1 (32, 166) -> (34.25, 166)
  line L2 (58, 396) -> (58, 166) projected
  line L3 (34.25, 166) -> (39.75, 166)
  line L4 (39.75, 166) -> (41, 166)
  line L5 (41, 166) -> (49.5, 166)
  line L6 (49.5, 166) -> (50.75, 166)
  line L7 (50.75, 166) -> (56.25, 166)
  line L8 (56.25, 166) -> (58, 166)
  line L9 (56.25, 166) -> (58, 166)
  line L10 (41, 166) -> (49.5, 166)
  line L11 (49.5, 166) -> (49.5, 140)
  line L12 (49.5, 140) -> (41, 140)
  line L13 (41, 140) -> (41, 166)
  line L14 (50.75, 166) -> (56.25, 166)
  line L15 (56.25, 166) -> (56.25, 140)
  line L16 (56.25, 140) -> (50.75, 140)
  line L17 (50.75, 140) -> (50.75, 166)
  line L18 (41, 166) -> (49.5, 166)
  line L19 (49.5, 166) -> (49.5, 396)
  line L20 (41, 396) -> (41, 166)
  line L21 (50.75, 166) -> (56.25, 166)
  line L22 (56.25, 166) -> (56.25, 396)
  line L23 (50.75, 396) -> (50.75, 166)
  line L24 (56.25, 396) -> (56.25, 396.25)
  line L25 (56.25, 396.25) -> (50.75, 396.25)
  line L26 (50.75, 396.25) -> (50.75, 396)
  line L27 (50.75, 396) -> (51, 396)
  line L28 (56.25, 396) -> (56, 396)
  arc A0 (51, 396.25) -> (50.75, 396) centre (51, 396) ccw
  arc A1 (56.25, 396) -> (56, 396.25) centre (56, 396) ccw
  arc A2 (54.25, 396) -> (52.75, 396) centre (53.5, 396) ccw
  line L29 (56.25, 396) -> (55.75, 396)
  line L30 (51.25, 396) -> (50.75, 396)
  line L31 (50.75, 396) -> (51.25, 396)
  line L32 (55.75, 396) -> (56.25, 396)
  line L33 (49.5, 396) -> (49.5, 396.25)
  line L34 (49.5, 396.25) -> (41, 396.25)
  line L35 (41, 396.25) -> (41, 396)
  line L36 (41, 396) -> (41.25, 396)
  line L37 (49.5, 396) -> (49.25, 396)
  arc A3 (41.25, 396.25) -> (41, 396) centre (41.25, 396) ccw
  arc A4 (49.5, 396) -> (49.25, 396.25) centre (49.25, 396) ccw
  line L38 (43.25, 396) -> (44.25, 396)
  line L39 (46.25, 396) -> (47.25, 396)
  line L40 (49, 396) -> (49.25, 396)
  arc A5 (44.4571, 396.25) -> (43.0429, 396.25) centre (43.75, 396) ccw
  arc A6 (47.4571, 396.25) -> (46.0429, 396.25) centre (46.75, 396) ccw
  line L41 (49.5, 396) -> (46, 396)
  line L42 (41, 396) -> (43, 396)
  line L43 (49, 396) -> (49.5, 396)
  line L44 (41.25, 396) -> (41.5, 396)
  line L45 (43, 396) -> (43.25, 396)
  line L46 (44.5, 396) -> (43, 396)
  line L47 (41.5, 396) -> (41, 396)
  line L48 (44.25, 396) -> (44.5, 396)
  line L49 (46, 396) -> (46.25, 396)
  point P0 (20, 0)
  point P1 (54.2071, 396.25)
  point P2 (52.7929, 396.25)
  dimension "d345" = 2.25
  dimension "d346" = 5.5
  dimension "d347" = 1.25
  dimension "d348" = 8.5
  dimension "d349" = 1.25
  dimension "d350" = 5.5
  dimension "d351" = 26
  dimension "d352" = 0.25
  dimension "d353" = 0.25
  dimension "d354" = 0.25
  dimension "d355" = 1.5
  dimension "d356" = 0.25
  dimension "d357" = 0.25
  dimension "d358" = 0.25
  dimension "d359" = 2
  dimension "d360" = 1
  dimension "d361" = 2
  dimension "d362" = 1
  dimension "d363" = 1.5
  constraints: 96 end point, 18 point on circle, 17 collinear, 17 parallel, 17 point on line, 10 perpendicular, 7 centre point, 5 midpoint, 4 coincident, 1 horizontal
  measures "d345" distance of L0.end L1.end
  measures "d346" distance of L1.end L3.end
  measures "d347" distance of L3.end L4.end
  measures "d348" distance of L4.end L5.end
  measures "d349" distance of L5.end L6.end
  measures "d350" distance of L6.end L7.end
  measures "d351" distance of L5.end L11.end
  measures "d352" distance of L24.end L22.end
  measures "d353" distance of L23.start L27.end
  measures "d354" distance of L22.end L28.end
  measures "d355" diameter of A2
  measures "d356" distance of L33.end L19.end
  measures "d357" distance of L20.start L36.end
  measures "d358" distance of L19.end L37.end
  measures "d359" distance of L44.start L38.start
  measures "d360" distance of L38.start L38.end
  measures "d361" distance of L38.end L39.start
  measures "d362" distance of L39.start L39.end
  measures "d363" diameter of A5
extrude "擠出19" cut sketch "草圖22" against normal blind 0.6 contours L20 A3 L34 A4 L19 L5 | L5 L11 L12 L13 | L23 A0 L25 A1 L22 L7 | L7 L15 L16 L17 | A5 L34 | L34 A6 | A2 L25